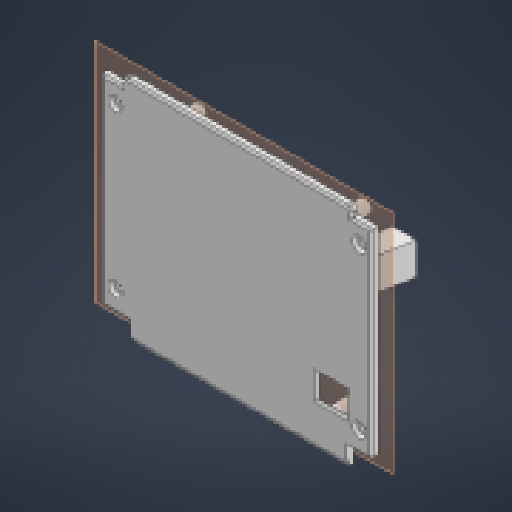
# Autodesk Inventor part: BP_BackCover
Saved by Autodesk Inventor 2026.1 (Build 301233020, 233B)
## iProperties
Created: 2025-09-13
Part Number: BP_BackCover
Material: Generic
Document SubType Name: Modeling
Designer: atrus
Density: 1 g/cm^3
Appearance: Default
Author: atrus
Autodesk Inventor part; units mm, degrees
ref_plane "YZ Plane" through (0, 0, 0) normal (1, 0, 0) x (0, 1, 0)
ref_plane "XZ Plane" through (0, 0, 0) normal (0, 1, 0) x (-1, 0, 0)
ref_plane "XY Plane" through (0, 0, 0) normal (0, 0, 1) x (1, 0, 0)
ref_plane "Work Plane1" through (0, 0, 0) normal (0, 0, 1) x (1, 0, 0)
sketch "Sketch1" plane through (0, 0, 0) normal (0, 0, 1) x (1, 0, 0)
  circle A0 centre (-111.199, -72) radius 2
  circle A1 centre (-5.483, -2.5) radius 2
  circle A2 centre (-111.199, -2.5) radius 2
  line L0 (-105.066, 0.2) -> (-96.966, 0.2)
  line L1 (-10.366, -5.012) -> (0, -5.012)
  line L2 (0, -5.012) -> (0, 5.5)
  line L3 (-9, 5.5) -> (0, 5.5)
  line L4 (-9, 5.5) -> (-9, 7.2)
  spline S0 degree 3 poles (-11.0328, 9.2) (-10.764, 9.2) (-10.4976, 9.1476) (-10.0026, 8.9441) (-9.7782, 8.7957) (-9.4033, 8.4236) (-9.2552, 8.2048) (-9.0524, 7.7216) (-9, 7.4622) (-9, 7.2) knots 0 0 0 0 0.253656 0.253656 0.505123 0.505123 0.752333 0.752333 1 1 1 1
  line L5 (-106.2992, 9.2) -> (-11.0328, 9.2)
  spline S1 degree 3 poles (-108.332, 7.2) (-108.332, 7.4565) (-108.2819, 7.7103) (-108.0866, 8.187) (-107.9426, 8.4048) (-107.577, 8.7772) (-107.3577, 8.9271) (-106.9875, 9.0869) (-106.8536, 9.1291) (-106.5792, 9.1857) (-106.4394, 9.2) (-106.2992, 9.2) knots 0 0 0 0 0.242386 0.242386 0.486827 0.486827 0.735395 0.735395 0.867613 0.867613 1 1 1 1
  line L6 (-108.332, 5.5) -> (-108.332, 7.2)
  line L7 (-117.332, 5.5) -> (-108.332, 5.5)
  line L8 (-117.332, -80) -> (-117.332, 5.5)
  line L9 (-105.066, -80) -> (-117.332, -80)
  line L10 (-105.066, -80) -> (-105.066, 0.2)
  circle A3 centre (-5.483, -72) radius 2
  line L11 (0, -19.352) -> (-10.366, -19.352)
  line L12 (-10.966, -79.0494) -> (-10.966, -80)
  line L13 (0, -80) -> (-10.966, -80)
  line L14 (0, -19.352) -> (0, -80)
  line L15 (0, -19.352) -> (0, -5.012)
  line L16 (-10.366, 2) -> (-10.366, -5.012)
  line L17 (-96.966, 0.2) -> (-96.966, 2)
  arc A4 (-93.166, 5.8) -> (-96.966, 2) centre (-93.166, 2) ccw
  line L18 (-93.166, 5.8) -> (-14.166, 5.8)
  arc A5 (-10.366, 2) -> (-14.166, 5.8) centre (-14.166, 2) ccw
  line L19 (-10.366, -19.352) -> (-10.366, -77)
  arc A6 (-10.966, -79.0494) -> (-10.366, -77) centre (-14.166, -77) ccw
  line L20 (-10.366, -19.352) -> (-10.366, -5.012)
  line L21 (-105.066, -80) -> (-104.866, -80)
  line L22 (-104.866, -80) -> (-104.866, -88.9)
  line L23 (-104.866, -88.9) -> (-11.166, -88.9)
  line L24 (-11.166, -88.9) -> (-11.166, -80)
  line L25 (-11.166, -80) -> (-10.966, -80)
  line L26 (-10.366, -73) -> (-105.066, -73)
  line L27 (-11.166, -86.9) -> (-104.866, -86.9) construction
  point P0 (0, 0)
  dimension "d0" = 0.2
  dimension "d1" = 0.2
  dimension "d2" = 2
  dimension "d3" = 7
  constraints: 16 end point, 4 perpendicular, 3 point on line, 2 horizontal, 1 vertical
  measures "d0" distance from line of L9.start L22
  measures "d1" distance from line of L12.end L24
  measures "d2" distance between parallel lines of L27 L23
  measures "d3" distance from line of L24.end L26
extrude "Extrusion1" add sketch "Sketch1" along normal blind 1.8 contours A0 | A1 | A2 | L10 L9 L8 L7 L6 S1 L5 S0 L4 L3 L2 L1 L16 A5 L18 A4 L17 L0 | L26 L19 A6 L12 L25 L24 L23 L22 L21 L10 | L19 L11 L14 L13 L12 A6 | L20 L1 L15 L11 | A3
sketch "Sketch2" plane through (0, 0, 1.8) normal (0, 0, 1) x (1, 0, 0)
  line L0 (0, -80) -> (0, 5.5) projected
  line L1 (0, 5.5) -> (-9, 5.5) projected
  line L2 (-9, 5.5) -> (-9, 7.2) projected
  ellipse E0 centre (-11.0328, 7.2) end of major axis (-9, 7.2) minor radius 2 (-9, 7.2) -> (-11.0328, 9.2) ccw projected
  line L3 (-11.0328, 9.2) -> (-106.2992, 9.2) projected
  ellipse E1 centre (-106.2992, 7.2) end of major axis (-104.2664, 7.1999) minor radius 2 (-106.2992, 9.2) -> (-108.332, 7.2) ccw projected
  line L4 (-108.332, 7.2) -> (-108.332, 5.5) projected
  line L5 (-108.332, 5.5) -> (-117.332, 5.5) projected
  line L6 (-117.332, 5.5) -> (-117.332, -80) projected
  line L7 (-117.332, -80) -> (-104.866, -80) projected
  line L8 (-104.866, -80) -> (-104.866, -88.9) projected
  line L9 (-104.866, -88.9) -> (-11.166, -88.9) projected
  line L10 (-11.166, -88.9) -> (-11.166, -80) projected
  line L11 (-11.166, -80) -> (0, -80) projected
  line L12 (-10.366, 2) -> (-10.366, -73) projected
  line L13 (-10.366, -73) -> (-105.066, -73) projected
  line L14 (-105.066, -73) -> (-105.066, 0.2) projected
  line L15 (-105.066, 0.2) -> (-96.966, 0.2) projected
  line L16 (-96.966, 0.2) -> (-96.966, 2) projected
  arc A0 (-93.166, 5.8) -> (-96.966, 2) centre (-93.166, 2) ccw projected
  line L17 (-93.166, 5.8) -> (-14.166, 5.8) projected
  arc A1 (-10.366, 2) -> (-14.166, 5.8) centre (-14.166, 2) ccw projected
  line L18 (-11.166, -86.9) -> (-104.866, -86.9) projected
  point P0 (0, 0)
  constraints: 2 other
extrude "Extrusion2" add sketch "Sketch2" along normal blind 1.2 contours L11 L10 L18 L8 L7 L6 L5 L4 E1 L3 E0 L2 L1 L0 | L12 L13 L14 L15 L16 A0 L17 A1
sketch "Sketch3" plane through (0, 0, 3) normal (0, 0, 1) x (1, 0, 0)
  line L0 (-11.166, -71) -> (-24.166, -71) projected
  line L1 (-11.166, -60) -> (-11.166, -71) projected
  line L2 (-24.166, -60) -> (-11.166, -60) projected
  line L3 (-24.166, -71) -> (-24.166, -60) projected
  line L4 (-24.166, -70.3) -> (-11.166, -70.3)
  point P0 (0, 0)
  dimension "d34" = 0.7
  constraints: 2 end point, 2 point on line, 1 horizontal
  measures "d34" distance between parallel lines of L0 L4
extrude "Extrusion3" cut sketch "Sketch3" against normal blind 3 contours L4 L3 L2 L1
sketch "Sketch4" plane through (0, 0, 3) normal (0, 0, 1) x (1, 0, 0)
  circle A0 centre (-5.483, -2.5) radius 2 construction
  circle A1 centre (-5.483, -72) radius 2 construction
  circle A2 centre (-111.199, -2.5) radius 2 construction
  circle A3 centre (-111.199, -72) radius 2 construction
  point P0 (0, 0)
  constraints: 4 coincident
hole "Hole1" at (-111.199, -72, 3) at (-111.199, -2.5, 3) at (-5.483, -2.5, 3) at (-5.483, -72, 3) direction (0, 0, -1) diameter 3.4 end through all counterbore diameter 6.3 counterbore depth 2 clearance for "Flat Head Machine Screw" size "M3" standard "Ansi Metric M Profile"
chamfer "Chamfer1" distance 1 angle 45 13 edges at (0, -37.25, 3) (-58.666, 9.2, 3) (-107.7366, 8.6142, 3) (-108.332, 6.35, 3) (-9.5954, 8.6142, 3) (-9, 6.35, 3) (-112.832, 5.5, 3) (-4.5, 5.5, 3) (-117.332, -37.25, 3) (-24.166, -65.15, 3) (-17.666, -60, 3) (-11.166, -65.15, 3) (-17.666, -70.3, 3)
sketch "Sketch5" plane through (0, 0, 0) normal (0, 0, -1) x (-1, 0, 0)
  line L0 (0, -19.352) -> (10.366, -19.352) projected
  line L1 (0, -80) -> (0, 5.5) projected
  line L2 (10.366, 2) -> (10.366, -73) projected
  line L3 (10.366, -5.012) -> (0, -5.012) projected
  line L4 (0, -19.152) -> (10.366, -19.152)
  line L5 (0, -5.212) -> (10.366, -5.212)
  point P0 (0, 0)
  dimension "d20" = 0.2
  dimension "d21" = 0.2
  constraints: 4 end point, 4 point on line, 2 perpendicular
  measures "d20" distance between parallel lines of L3 L5
  measures "d21" distance between parallel lines of L0 L4
extrude "Extrusion4" add sketch "Sketch5" along normal blind 8 contours L1 L5 L2 L4
sketch "Sketch7" plane through (-10.366, -5.212, 0) normal (0, 1, 0) x (1, 0, 0)
  line L0 (10.366, 0) -> (10.366, 8) projected
  line L1 (0, 13.9798) -> (12.7429, 13.9798) projected
  line L2 (0, 8) -> (10.366, 8) projected
  line L3 (0, 0) -> (0, 13.6) projected
  line L4 (2, 13.9798) -> (2, 8)
  line L5 (2, 13.7798) -> (12.7859, 13.7798)
  spline S0 degree 3 poles (1.366, 54.07) (2.6114, 54.07) (3.9309, 53.8595) (6.2483, 52.8955) (7.2365, 52.2155) (8.6015, 50.9016) (9.0798, 50.326) (10.3635, 48.5092) (10.9891, 47.2127) (11.8316, 45.0211) (12.1129, 44.127) (12.7735, 41.6602) (13.0681, 40.0838) (13.5276, 36.7721) (13.6742, 35.0374) (13.8523, 31.3701) (13.8669, 29.4389) (13.7666, 24.7854) (13.5948, 22.0679) (13.041, 16.0946) (12.6224, 12.8476) (11.6152, 6.396) (11.0258, 3.1892) (10.366, 0) knots 0 0 0 0 0.309903 0.309903 0.584179 0.584179 0.77016 0.77016 1.152617 1.152617 1.413042 1.413042 1.86998 1.86998 2.374169 2.374169 2.940222 2.940222 3.743245 3.743245 4.712988 4.712988 5.681003 5.681003 5.681003 5.681003 projected
  point P0 (12.7169, 13.7798)
  dimension "d24" = 0.2
  dimension "d25" = 2
  constraints: 4 end point, 3 point on line, 1 perpendicular, 1 vertical
  measures "d24" distance between parallel lines of L1 L5
  measures "d25" distance between parallel lines of L3 L4
extrude "Extrusion5" add sketch "Sketch7" against normal up to surface (13.94 mm away) contours L0 L2 L4 L5 S0
sketch "Sketch8" plane through (0, 0, 1.8) normal (0, 0, -1) x (-1, 0, 0)
  circle A0 centre (17.916, -73.25) radius 1.8 projected
  circle A1 centre (17.916, -73.25) radius 1.8 projected
  circle A2 centre (17.916, -1.75) radius 1.8 projected
  circle A3 centre (89.416, -1.75) radius 1.8 projected
  circle A4 centre (89.416, -73.25) radius 1.8 projected
  circle A5 centre (89.416, -1.75) radius 2.8
  circle A6 centre (17.916, -1.75) radius 2.8
  circle A7 centre (17.916, -73.25) radius 2.8
  circle A8 centre (89.416, -73.25) radius 2.8
  point P0 (0, 0)
  dimension "d28" = 1
  dimension "d29" = 1
  dimension "d30" = 1
  dimension "d31" = 1
  constraints: 4 centre point, 2 coincident
  measures "d28" radial gap between concentric circles of A8 A4
  measures "d29" radial gap between concentric circles of A7 A0
  measures "d30" radial gap between concentric circles of A6 A2
  measures "d31" radial gap between concentric circles of A5 A3
ref_plane "Work Plane2" through (-96.166, -80, -11.9798) normal (0, 0, 1) x (1, 0, 0)
extrude "Extrusion6" add sketch "Sketch8" along normal up to surface (13.7798 mm away)
body "Solid1"
